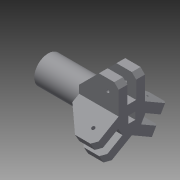
# Autodesk Inventor part: Coupler
Saved by Autodesk Inventor 2014 SP1 (Build 180222100, 222)
## iProperties
Created: 2014-01-24
Part Number: Coupler
Material: Generic
Document SubType Name: Modeling
Designer: tom
Density: 1 g/cm^3
Appearance: Default
Author: tom
Autodesk Inventor part; units mm, degrees
ref_plane "YZ Plane" through (0, 0, 0) normal (1, 0, 0) x (0, 1, 0)
ref_plane "XZ Plane" through (0, 0, 0) normal (0, 1, 0) x (-1, 0, 0)
ref_plane "XY Plane" through (0, 0, 0) normal (0, 0, 1) x (1, 0, 0)
sketch "Sketch1" plane through (0, 0, 0) normal (1, 0, 0) x (0, 1, 0)
  circle A0 centre (0, 0) radius 3.175
  circle A1 centre (0, 0) radius 6.35
  dimension "d0" = 6.35
  dimension "d1" = 12.7
  constraints: 2 centre point, 2 coincident
  measures "d0" diameter of A0
  measures "d1" diameter of A1
extrude "Extrusion1" add sketch "Sketch1" along normal blind 25.4
sketch "Sketch2" plane through (25.4, 0, 0) normal (1, 0, 0) x (0, 0, -1)
  circle A0 centre (0, 0) radius 6.35 projected
  circle A1 centre (0, 0) radius 1.5875
  circle A2 centre (0, 0) radius 6.35
  dimension "d4" = 3.175
  constraints: 2 centre point, 2 coincident, 1 concentric
  measures "d4" diameter of A1
extrude "Extrusion2" add sketch "Sketch2" along normal blind 12.7
sketch "Sketch3" plane through (38.1, 0, 0) normal (1, 0, 0) x (0, 0, -1)
  circle A0 centre (0, 0) radius 6.35 projected
  line L0 (2, 16.0268) -> (2, 6.0268)
  line L1 (2, 16.0268) -> (6, 16.0268)
  line L2 (6, 16.0268) -> (6, 2.0791)
  line L3 (-2, 16.0268) -> (-2, 6.0268)
  line L4 (-2, 16.0268) -> (-6, 16.0268)
  line L5 (-6, 16.0268) -> (-6, 2.0791)
  dimension "d11" = 4
  dimension "d12" = 10
  dimension "d13" = 10
  constraints: 12 end point, 4 perpendicular, 4 point on circle
  measures "d11" distance of L3.start L4.end
  measures "d12" distance of L0.end L0.start
  measures "d13" distance of L3.end L3.start
extrude "Extrusion3" add sketch "Sketch3" against normal blind 18 contours A0 L0 L1 L2 | L5 L4 L3 A0
chamfer "Chamfer1" distance 9 angle 45 2 edges at (20.1, 16.0268, 4) (20.1, 16.0268, -4)
chamfer "Chamfer2" distance 2 angle 45 2 edges at (38.1, 16.0268, 4) (38.1, 16.0268, -4)
sketch "Sketch5" plane through (20.1, 2.0791, 6) normal (0, 0, 1) x (1, 0, 0)
  line L0 (16, 13.9478) -> (9, 13.9478) projected
  line L1 (18, 11.9478) -> (18, 0) projected
  circle A0 centre (13, 8.9478) radius 0.75
  point P0 (-20.1, -2.0791)
  dimension "d30" = 1.5
  dimension "d31" = 5
  dimension "d32" = 5
  constraints: 1 centre point
  measures "d30" diameter of A0
  measures "d31" distance from line of L0 A0.centre
  measures "d32" distance from line of A0.centre L1
extrude "Extrusion5" cut sketch "Sketch5" against normal blind 15
sketch "Sketch6" plane through (38.1, 0, 0) normal (1, 0, 0) x (0, 0, -1)
  arc A0 (2, 6.0268) -> (-2, 6.0268) centre (0, 0) ccw projected
  line L0 (-6, 14.0268) -> (-6, 2.0791) projected
  line L1 (2, 6.0268) -> (-2, 6.0268)
  point P0 (-6, 3.4641)
  constraints: 2 end point, 1 perpendicular, 1 point on circle
extrude "Extrusion6" cut sketch "Sketch6" against normal blind 6
pattern_circular "Circular Pattern3" count 3 over 360 about axis through (0, 0, 0) along (1, 0, 0) of "Extrusion3", "Chamfer2", "Extrusion5", "Extrusion6", "Chamfer1"
sketch "Sketch7" plane through (38.1, 0, 0) normal (1, 0, 0) x (0, 0, -1)
  circle A0 centre (0, 0) radius 1.5875 projected
  circle A1 centre (0, 0) radius 1.524
  line L0 (-1.524, 1.524) -> (1.524, 1.524)
  line L1 (1.524, 1.524) -> (1.524, -1.524)
  line L2 (1.524, -1.524) -> (-1.524, -1.524)
  line L3 (-1.524, -1.524) -> (-1.524, 1.524)
  circle A2 centre (0, 0) radius 1.5875
  dimension "d43" = 3.048
  constraints: 8 end point, 2 centre point, 2 coincident, 2 parallel, 1 concentric, 1 horizontal, 1 perpendicular
  measures "d43" diameter of A1
extrude "Extrusion7" add sketch "Sketch7" against normal blind 3.175 contours A0 L1 | L1 A1 L0 A0 | A0 L2 A1 L1 | L0 A0 | A1 | A0 L2 | L0 A1 L3 A0 | L2 A0 L3 A1 | L3 A0
sketch "Sketch8" plane through (38.1, 0, 0) normal (1, 0, 0) x (0, 0, -1)
  line L0 (-1.651, 1.651) -> (1.651, 1.651)
  line L1 (1.651, 1.651) -> (1.651, -1.651)
  line L2 (1.651, -1.651) -> (-1.651, -1.651)
  line L3 (-1.651, -1.651) -> (-1.651, 1.651)
  point P0 (0, 0)
  dimension "d46" = 1.651
  dimension "d48" = 1.651
  dimension "d49" = 3.302
  dimension "d50" = 3.302
  constraints: 8 end point, 2 parallel, 1 horizontal, 1 perpendicular
  measures "d46" horizontal distance of L0.start point (0, 0)
  measures "d48" distance from line of point (0, 0) L3
  measures "d49" distance of L0.end L1.end
  measures "d50" distance of L1.end L2.end
extrude "Extrusion8" cut sketch "Sketch8" against normal blind 12.7
body "Solid1"
